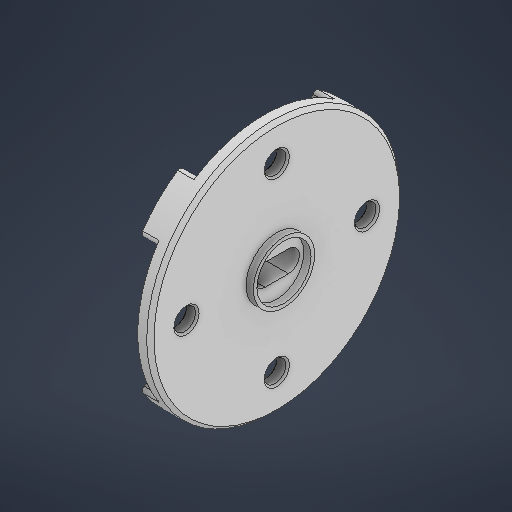
# Autodesk Inventor part: Wheel_Hub_V2
Saved by Autodesk Inventor 2026.1 (Build 301233000, 233)
## iProperties
Created: 2026-09-11
Part Number: Wheel_Hub_V2
Material: Generic
Document SubType Name: Modeling
Designer: share
Density: 1 g/cm^3
Appearance: Default
Author: share
Autodesk Inventor part; units mm, degrees
ref_plane "YZ Plane" through (0, 0, 0) normal (1, 0, 0) x (0, 1, 0)
ref_plane "XZ Plane" through (0, 0, 0) normal (0, 1, 0) x (-1, 0, 0)
ref_plane "XY Plane" through (0, 0, 0) normal (0, 0, 1) x (1, 0, 0)
sketch "Sketch1" plane through (0, 0, 0) normal (1, 0, 0) x (0, 1, 0)
  circle A0 centre (0, 0) radius 70
  dimension "d0" = 140
  constraints: 1 centre point, 1 coincident
  measures "d0" diameter of A0
extrude "Extrusion1" add sketch "Sketch1" along normal blind 7
sketch "Sketch2" plane through (7, 0, 0) normal (1, 0, 0) x (0, 0, -1)
  circle A0 centre (0, 0) radius 50 construction
  line L0 (0, 0) -> (0, 50) construction
  dimension "d3" = 100
  constraints: 2 coincident, 2 end point, 1 vertical, 1 vertical alignment, 2 other
hole "Hole1" at (7, 50, 0) direction (-1, 0, 0) diameter 12 end through all
pattern_circular "Circular Pattern1" count 4 over 360 about axis through (-10, 0, 0) along (1, 0, 0) of "Hole1"
sketch "Sketch4" plane through (7, 0, 0) normal (1, 0, 0) x (0, 0, -1)
  circle A0 centre (0, 0) radius 15
  circle A1 centre (0, 0) radius 17
  dimension "d19" = 30
  dimension "d20" = 34
  constraints: 2 centre point, 2 coincident
  measures "d19" diameter of A0
  measures "d20" diameter of A1
extrude "Extrusion3" add sketch "Sketch4" along normal blind 4
sketch "Sketch5" plane through (0, 0, 0) normal (-1, 0, 0) x (0, 0, 1)
  line L0 (-98, 0) -> (98, 0) construction
  line L1 (0, 98) -> (0, -98) construction
  line L2 (0, 0) -> (49.497475, 49.497475) construction
  circle A0 centre (0, 0) radius 70
  circle A1 centre (0, 0) radius 70
  circle A2 centre (0, 0) radius 55
  dimension "d23" = 45
  dimension "d25" = 140
  dimension "d26" = 110
  constraints: 2 centre point, 2 coincident, 2 end point, 2 other
  measures "d23" angle of L0 L2
  measures "d25" diameter of A1
  measures "d26" diameter of A2
extrude "Extrusion4" add sketch "Sketch5" along normal blind 9
sketch "Sketch6" plane through (-9, 0, 0) normal (-1, 0, 0) x (0, 0, 1)
  circle A0 centre (0, 0) radius 70
  circle A1 centre (0, 0) radius 55
  line L0 (-98, 0) -> (98, 0) construction
  line L1 (0, 104) -> (0, -99) construction
  arc A2 (-36.874788, 59.5) -> (36.874788, 59.5) centre (0, 75) ccw
  point P0 (28.565714, 47)
  point P1 (-28.565714, 47)
  dimension "d29" = 75
  dimension "d30" = 40
  constraints: 4 point on circle, 1 centre point, 1 point on line
  measures "d29" distance from line of L0 A2.centre
  measures "d30" radius of A2
extrude "Extrusion5" cut sketch "Sketch6" against normal up to surface (9 mm away) contours A2 A1 A0 picked at (-26.152948, 55.591965)
pattern_circular "Circular Pattern2" count 4 over 360 about axis through (-10, 0, 0) along (1, 0, 0) of "Extrusion5"
sketch "Sketch7" plane through (-9, 0, 0) normal (-1, 0, 0) x (0, 0, 1)
  circle A0 centre (0, 0) radius 62.5 construction
  line L0 (-98, 0) -> (98, 0) construction
  line L1 (0, 98) -> (0, -98) construction
  line L2 (0, 0) -> (44.194174, 44.194174) construction
  dimension "d36" = 125
  dimension "d37" = 45
  constraints: 2 coincident, 2 end point, 3 other
  measures "d37" angle of L1 L2
hole "Hole2" at (-9, 44.194174, 44.194174) direction (1, 0, 0) diameter 9.144 depth 10 tip angle 118 thread size "7/16-14 UNC" class "2B" standard "ANSI Unified Screw Threads"
pattern_circular "Circular Pattern3" count 4 over 360 about axis through (-10, 0, 0) along (1, 0, 0) of "Hole2"
fillet "Fillet2" radius 2 16 edges at (-4.5, 59.5, 36.8748) (-4.5, 59.5, -36.8748) (-4.5, 47, 28.5657) (-4.5, 47, -28.5657) (-4.5, 28.5657, 47) (-4.5, -28.5657, 47) (-4.5, 36.8748, 59.5) (-4.5, -36.8748, 59.5) (-4.5, -47, -28.5657) (-4.5, -47, 28.5657) (-4.5, -59.5, -36.8748) (-4.5, -59.5, 36.8748) (-4.5, 28.5657, -47) (-4.5, -28.5657, -47) (-4.5, 36.8748, -59.5) (-4.5, -36.8748, -59.5)
sketch "Sketch8" plane through (0, 0, 0) normal (-1, 0, 0) x (0, 0, 1)
  circle A0 centre (0, 0) radius 15
  circle A1 centre (0, 0) radius 22.5
  line L0 (6.5, -6) -> (-6.5, -6) projected
  arc A2 (6.5, -6) -> (6.5, 6) centre (6.5, 0) ccw projected
  line L1 (12.5, 1.5) -> (12.5, -1.5) projected
  arc A3 (6.5, -6) -> (6.5, 6) centre (6.5, 0) ccw projected
  line L2 (-6.5, 6) -> (6.5, 6) projected
  arc A4 (-6.5, 6) -> (-6.5, -6) centre (-6.5, 0) ccw projected
  line L3 (-12.5, -1.5) -> (-12.5, 1.5) projected
  arc A5 (-6.5, 6) -> (-6.5, -6) centre (-6.5, 0) ccw projected
  dimension "d49" = 30
  dimension "d50" = 45
  constraints: 2 centre point, 2 coincident
  measures "d49" diameter of A0
  measures "d50" diameter of A1
extrude "Extrusion6" add sketch "Sketch8" along normal blind 20 contours A0 | A1 | L0 A4 L2 A2
chamfer "Chamfer1" distance 2 angle 45 1 edges at (7, -70, 0)
chamfer "Chamfer2" distance 1 angle 45 8 edges at (0, 6, -50) (0, 50, 6) (0, -6, 50) (0, -50, -6) (7, 50, 6) (7, -6, 50) (7, 6, -50) (7, -50, -6)
sketch "Sketch3" plane through (7, 0, 0) normal (1, 0, 0) x (0, 0, -1)
  line L0 (-98, 0) -> (98, 0) construction
  line L1 (0, -98) -> (0, 98) construction
  line L2 (-12.5, 6) -> (12.5, 6)
  line L3 (12.5, 6) -> (12.5, -6)
  line L4 (12.5, -6) -> (-12.5, -6)
  line L5 (-12.5, -6) -> (-12.5, 6)
  point P0 (0, 0)
  dimension "d14" = 25
  dimension "d15" = 12
  constraints: 8 end point, 2 parallel, 1 horizontal, 1 perpendicular, 2 other
  measures "d14" distance between parallel lines of L3 L5
  measures "d15" distance between parallel lines of L4 L2
extrude "Extrusion7" cut sketch "Sketch3" against normal up to surface (27 mm away)
fillet "Fillet3" radius 6 4 edges at (-6.5, 6, -12.5) (-6.5, -6, -12.5) (-6.5, -6, 12.5) (-6.5, 6, 12.5)
body "Solid1"
